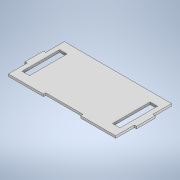
# Autodesk Inventor part: Level2 (Arduino)
Saved by Autodesk Inventor 2020 (Build 240168000, 168)
## iProperties
Created: 2020-01-30
Part Number: Level2 (Arduino)
Material: Generic
Document SubType Name: Modeling
Designer: jelte
Density: 1 g/cm^3
Appearance: Default
Mass: 27.8577 g
Surface Area: 213.03 cm^2
Volume: 27.8577 cm^3
Author: jelte
Autodesk Inventor part; units mm, degrees
ref_plane "YZ Plane" through (0, 0, 0) normal (1, 0, 0) x (0, 1, 0)
ref_plane "XZ Plane" through (0, 0, 0) normal (0, 1, 0) x (-1, 0, 0)
ref_plane "XY Plane" through (0, 0, 0) normal (0, 0, 1) x (1, 0, 0)
sketch "Sketch1" plane through (0, 0, 0) normal (0, 1, 0) x (-1, 0, 0)
  line L0 (71.1097, -38.0648) -> (71.1097, -13.0648)
  line L1 (71.1097, -13.0648) -> (74.1097, -13.0648)
  line L2 (74.1097, -13.0648) -> (74.1097, 11.9352)
  line L3 (74.1097, 11.9352) -> (71.1097, 11.9352)
  line L4 (71.1097, 11.9352) -> (71.1097, 36.9352)
  line L5 (-72.8903, -38.0648) -> (-72.8903, -13.0648)
  line L6 (-72.8903, 36.9352) -> (-72.8903, 11.9352)
  line L7 (-72.8903, -13.0648) -> (-75.8903, -13.0648)
  line L8 (-75.8903, -13.0648) -> (-75.8903, 11.9352)
  line L9 (-75.8903, 11.9352) -> (-72.8903, 11.9352)
  line L10 (71.1097, -38.0648) -> (-72.8903, -38.0648)
  line L11 (71.1097, 36.9352) -> (-72.8903, 36.9352)
  point P0 (0, 0)
  constraints: 24 end point, 5 perpendicular, 3 horizontal, 2 vertical
extrude "Extrusion1" add sketch "Sketch1" along normal blind 3
sketch "Sketch2" plane through (0, 3, 0) normal (0, 1, 0) x (1, 0, 0)
  line L0 (-74.1097, 13.0648) -> (-74.1097, -11.9352) projected
  line L1 (75.8903, -11.9352) -> (75.8903, 13.0648) projected
  line L2 (-71.1097, -36.9352) -> (72.8903, -36.9352) projected
  line L3 (-24.1097, -36.9352) -> (25.8903, -36.9352)
  line L4 (25.8903, -36.9352) -> (25.8903, -33.9352)
  line L5 (25.8903, -33.9352) -> (-24.1097, -33.9352)
  line L6 (-24.1097, -33.9352) -> (-24.1097, -36.9352)
  line L7 (72.8903, 38.0648) -> (-71.1097, 38.0648) projected
  point P0 (0, 0)
  dimension "d13" = 50
  dimension "d14" = 3
  constraints: 8 end point, 2 parallel, 1 horizontal, 1 perpendicular, 1 point on line
  measures "d13" distance of L4.end L5.end
  measures "d14" distance of L3.end L4.end
extrude "Extrusion2" cut sketch "Sketch2" against normal blind 30
sketch "Sketch3" plane through (0, 3, 0) normal (0, 1, 0) x (1, 0, 0)
  line L0 (-71.1097, -36.9352) -> (-24.1097, -36.9352) projected
  line L1 (-74.1097, 13.0648) -> (-74.1097, -11.9352) projected
  line L2 (-54.9097, 25.4648) -> (-64.9114, 25.4648)
  line L3 (-64.9114, 25.4648) -> (-64.9114, -24.8352)
  line L4 (-64.9114, -24.8352) -> (-54.9097, -24.8352)
  line L5 (-54.9097, -24.8352) -> (-54.9097, 25.4648)
  line L6 (56.6903, 25.4648) -> (66.6903, 25.4648)
  line L7 (66.6903, 25.4648) -> (66.6903, -24.8352)
  line L8 (66.6903, -24.8352) -> (56.6903, -24.8352)
  line L9 (56.6903, -24.8352) -> (56.6903, 25.4648)
  circle A0 centre (-34.6697, 22.9248) radius 2
  circle A1 centre (-35.9397, -22.2952) radius 2
  circle A2 centre (40.2603, 22.9248) radius 2
  circle A3 centre (46.6103, -22.2952) radius 2
  line L10 (-49.9097, 28.4648) -> (51.6903, 28.4648)
  line L11 (51.6903, 28.4648) -> (51.6903, 33.4648)
  line L12 (51.6903, 33.4648) -> (-49.9097, 33.4648)
  line L13 (-49.9097, 33.4648) -> (-49.9097, 28.4648)
  point P0 (0, 0)
  dimension "d32" = 4
  dimension "d35" = 4
  dimension "d38" = 4
  dimension "d39" = 4
  constraints: 24 end point, 6 parallel, 4 centre point, 3 horizontal, 3 perpendicular
  measures "d32" diameter of A0
  measures "d35" diameter of A1
  measures "d38" diameter of A2
  measures "d39" diameter of A3
extrude "Extrusion3" cut sketch "Sketch3" against normal blind 10
sketch "Sketch4" plane through (0, 3, 0) normal (0, 1, 0) x (1, 0, 0)
  circle A0 centre (-34.6697, 22.9248) radius 2 projected
  circle A1 centre (-34.6697, 22.9248) radius 2
  circle A2 centre (40.2603, 22.9248) radius 2 projected
  circle A3 centre (40.2603, 22.9248) radius 2
  circle A4 centre (46.6103, -22.2952) radius 2 projected
  circle A5 centre (46.6103, -22.2952) radius 2
  circle A6 centre (-35.9397, -22.2952) radius 2 projected
  circle A7 centre (-35.9397, -22.2952) radius 2
  point P0 (0, 0)
  constraints: 4 centre point, 4 coincident
extrude "Extrusion4" add sketch "Sketch4" against normal blind 3
sketch "Sketch5" plane through (-49.9097, 3, -28.4648) normal (1, 0, 0) x (0, 0, -1)
  line L0 (0, 0) -> (5, 0) projected
  line L1 (0, 0) -> (5, 0)
  line L2 (5, 0) -> (5, -3)
  line L3 (5, -3) -> (0, -3)
  line L4 (0, -3) -> (0, 0)
  point P0 (-28.4648, -3)
  constraints: 8 end point, 2 parallel, 1 horizontal, 1 perpendicular
extrude "Extrusion5" add sketch "Sketch5" along normal blind 102.075
body "Solid1"
